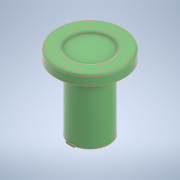
# Autodesk Inventor part: BOTÃO
Saved by Autodesk Inventor 2022 (Build 260153000, 153)
## iProperties
Created: 2023-07-20
Part Number: BOTÃO
Material: Generic
Document SubType Name: Modeling
Designer: Usuário
Density: 1 g/cm^3
Appearance: Red
Author: Usuário
Autodesk Inventor part; units mm, degrees
ref_plane "YZ Plane" through (0, 0, 0) normal (1, 0, 0) x (0, 1, 0)
ref_plane "XZ Plane" through (0, 0, 0) normal (0, 1, 0) x (-1, 0, 0)
ref_plane "XY Plane" through (0, 0, 0) normal (0, 0, 1) x (1, 0, 0)
sketch "Sketch2" plane through (0, 0, 0) normal (1, 0, 0) x (0, 1, 0)
  line L0 (0, 0) -> (-4, 0)
  line L1 (-4, 0) -> (-4, -12.5)
  line L2 (-4, -12.5) -> (0, -12.5)
  line L3 (0, -12.5) -> (0, 0)
  line L4 (12.3022, 0) -> (-32.9738, 0) construction
  line L5 (-4, 0) -> (-28, 0)
  line L6 (-28, 0) -> (-28, -7)
  line L7 (-28, -7) -> (-4, -7)
  line L8 (-4, -7) -> (-4, 0)
  line L9 (-4, -6) -> (-28, -6)
  point P0 (-4, -7)
  dimension "d0" = 4
  dimension "d2" = 25
  dimension "d3" = 28
  dimension "d4" = 1
  dimension "d5" = 14
  constraints: 20 end point, 4 horizontal, 4 parallel, 2 perpendicular, 2 point on line
  measures "d0" distance of L2.end L1.end
  measures "d2" diameter of L2 L4
  measures "d3" distance between parallel lines of L6 L3
  measures "d4" distance between parallel lines of L7 L9
  measures "d5" diameter of L7 L4
revolve "Revolution1" add sketch "Sketch2" angle 360 about axis through (0, 12.3022, 0) along (0, -1, 0) contours L3 L2 L1 L0 | L1 L7 L6 L9
sketch "Sketch3" plane through (0, 0, 0) normal (0, 1, 0) x (1, 0, 0)
  circle A0 centre (0, 0) radius 7
  dimension "d7" = 14
  constraints: 1 centre point
  measures "d7" diameter of A0
extrude "Extrusion1" cut sketch "Sketch3" against normal blind 1
fillet "Fillet1" radius 2 1 edges at (-7, 0, 0)
fillet "Fillet2" radius 1 1 edges at (0, 0, 12.5)
sketch "Sketch4" plane through (0, -28, 0) normal (0, -1, 0) x (1, 0, 0)
  circle A0 centre (0, 0) radius 7 projected
  circle A1 centre (0, 0) radius 7 projected
  line L0 (1.5845, 7.3307) -> (1.5845, 6.8183)
  line L1 (1.5845, -6.8183) -> (1.5845, -7.3307)
  line L2 (-1.5845, 7.3307) -> (-1.5845, 6.8183)
  line L3 (-1.5845, -6.8183) -> (-1.5845, -7.3307)
  circle A2 centre (0, 0) radius 11.5 projected
  arc A3 (1.5845, 7.3307) -> (-1.5845, 7.3307) centre (0, 0) ccw
  arc A4 (-1.5845, -7.3307) -> (1.5845, -7.3307) centre (0, 0) ccw
  dimension "d13" = 1.5845
  dimension "d14" = 1.5845
  dimension "d15" = 1.5845
  dimension "d16" = 1.5845
  constraints: 8 end point, 8 point on circle, 4 parallel, 2 centre point, 2 vertical
  measures "d13" horizontal distance of A2.centre L1.start
  measures "d14" distance from line of L3 point (0, 0)
  measures "d15" horizontal distance of L0.start point (0, 0)
  measures "d16" horizontal distance of L2.end point (0, 0)
extrude "Extrusion2" add sketch "Sketch4" against normal blind 0.5 contours A0 L2 A3 L0 | L1 A4 L3 A0
body "Solid1"
